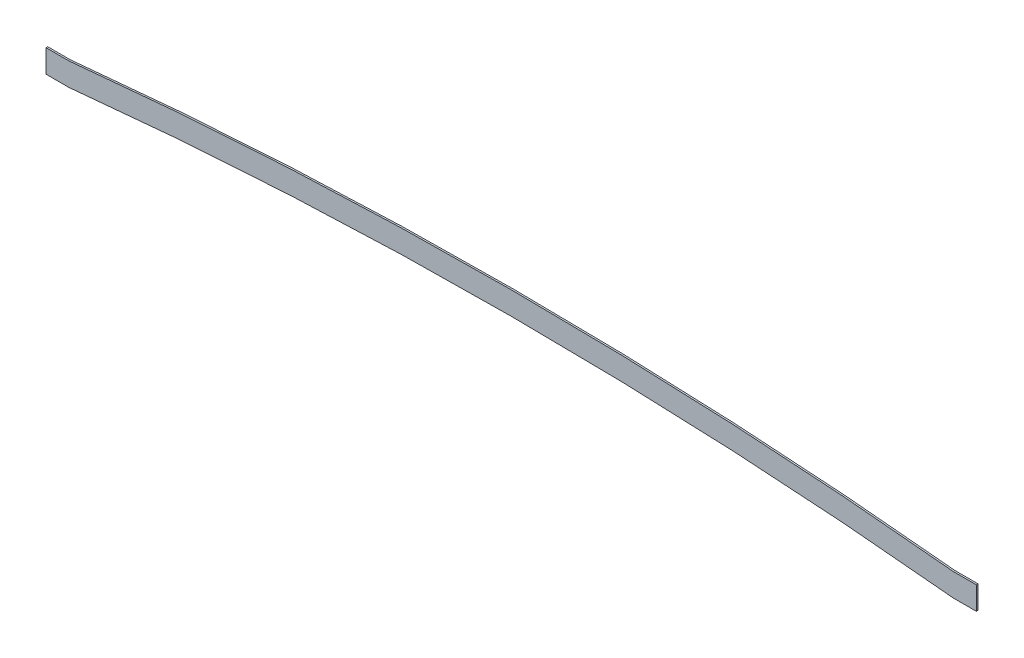
# Autodesk Inventor part: МОО 041 шпангоут спина 1
Saved by Autodesk Inventor 2024.2 (Build 282272000, 272)
## iProperties
Created: 2024-04-28
Part Number: МОО 041 шпангоут спина 1
Material: Generic
Document SubType Name: Sheet Metal
Designer: admin
Density: 1 g/cm^3
Sheet Metal Rule: Default_mm
Appearance: Default
Author: admin
Autodesk Inventor part; units mm, degrees
ref_plane "YZ Plane" through (0, 0, 0) normal (1, 0, 0) x (0, 1, 0)
ref_plane "XZ Plane" through (0, 0, 0) normal (0, 1, 0) x (-1, 0, 0)
ref_plane "XY Plane" through (0, 0, 0) normal (0, 0, 1) x (1, 0, 0)
sketch "Sketch1" plane through (0, 0, 0) normal (0, 0, 1) x (1, 0, 0)
  line L0 (-770, 40) -> (770, 40) construction
  line L1 (770, 40) -> (770, 0) construction
  line L2 (770, -40) -> (-770, -40) construction
  line L3 (-770, -40) -> (-770, 0)
  line L4 (-770, 0) -> (770, 0) construction
  line L5 (-770, 0) -> (-770, 40) construction
  line L6 (770, 0) -> (770, -40)
  arc A0 (770, -40) -> (-770, -40) centre (0, -7431.25) ccw
  arc A1 (770, 0) -> (-770, 0) centre (0, -7391.25) ccw
  line L7 (-770, 0) -> (-810, 0)
  line L8 (-810, 0) -> (-810, -40)
  line L9 (-810, -40) -> (-770, -40)
  line L10 (770, 0) -> (810, 0)
  line L11 (810, 0) -> (810, -40)
  line L12 (810, -40) -> (770, -40)
  point P0 (0, 0)
  point P1 (0, 0)
  dimension "d0" = 80
  dimension "d1" = 40
  dimension "d2" = 1620
  measures "d0" distance of L1.start L6.end
  measures "d1" distance of L4.start L7.end
  measures "d2" distance between parallel lines of L11 L8
extrude "Plate1" add sketch "Sketch1" along normal blind 3
equation "\"d0\" = 2 * d3"
equation "\"d1\" = d3"
equation "\"d2\" = d4 - d0"
equation "\"d5\" = Thickness"
equation "\"BendRadius\" = Thickness"
equation "\"BendReliefWidth\" = Thickness"
equation "\"BendReliefDepth\" = 0.5 * Thickness"
equation "\"CornerReliefSize\" = 4 * Thickness"
equation "\"MinimumRemnant\" = 2 * Thickness"
equation "\"TransitionRadius\" = BendRadius"
equation "\"JacobiRadiusSize\" = BendRadius"
equation "\"GapSize\" = Thickness"
equation "\"d3\" = 40"
equation "\"d4\" = 1700"
equation "\"Thickness\" = 3"
body "Solid1"
